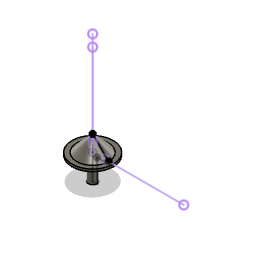
electrode V2 Al in Ni Dipper v1 (Autodesk Fusion 360 design; units mm, degrees)
Autodesk Fusion 360 part; units mm, degrees
sketch "Skizze1" plane through (0, 0, 0) normal (0, 0, 1) x (1, 0, 0)
  line L0 (3.5, 0) -> (4.5, 0)
  line L1 (3.5, 0) -> (0, 3.5)
  line L2 (0, 1.75) -> (0, 22.5)
  line L3 (20, 0) -> (2.5, 0)
  line L4 (4.5, 0) -> (4.5, -0.5)
  line L5 (0, 2.5) -> (0, 20)
  line L6 (0.95, -0.5) -> (4.5, -0.5)
  line L7 (0.95, -0.5) -> (0.95, -5.5)
  line L8 (0.95, -5.5) -> (0, -5.5)
  line L9 (0, -5.5) -> (0, 3.5)
  point P0 (0.95, -0.5)
  dimension "d7" = 1
  dimension "d8" = 3.5
  dimension "d11" = 45
  dimension "d12" = 0.5
  dimension "d13" = 0.95
  dimension "d14" = 0.5
  dimension "d15" = 5
  constraint horizontal L0
  constraint coincident L1.end L2
  constraint coincident L0.start L3
  constraint perpendicular L0 L4
  constraint coincident P0 L6.start
  constraint perpendicular L6 L7
  constraint perpendicular L7 L8
  constraint parallel L5 L9
  measures "d7" distance of L0.start L0.end
  measures "d8" distance of origin L0.start
  measures "d11" angle of L1 L3
  measures "d12" distance of L0.end L4.end
  measures "d13" distance of P0 L5
  measures "d14" distance of L3 P0
  measures "d15" distance of P0 L7.end
revolve "Drehen2" add sketch "Skizze1" angle 360 about axis through (0, -5.5, 0) along (0, 1, 0)
equation "d13 = ( 1.9 / 2 ) * 1 mm"
